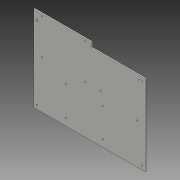
# Autodesk Inventor part: Plate-0
Saved by Autodesk Inventor 2018 (Build 220112000, 112)
## iProperties
Created: 2022-04-19
Part Number: Plate-0
Material: Generic
Document SubType Name: Modeling
Designer: pollak
Density: 1 g/cm^3
Appearance: Default
Author: pollak
Autodesk Inventor part; units mm, degrees
ref_plane "YZ Plane" through (0, 0, 0) normal (1, 0, 0) x (0, 1, 0)
ref_plane "XZ Plane" through (0, 0, 0) normal (0, 1, 0) x (-1, 0, 0)
ref_plane "XY Plane" through (0, 0, 0) normal (0, 0, 1) x (1, 0, 0)
sketch "Sketch1" plane through (0, 0, 0) normal (0, 1, 0) x (-1, 0, 0)
  line L0 (135, 97.5) -> (-135, 97.5)
  line L1 (-135, 97.5) -> (-135, -97.5)
  line L2 (-135, -97.5) -> (135, -97.5)
  line L3 (135, -97.5) -> (135, 97.5)
  line L4 (135, 97.5) -> (-135, -97.5) construction
  line L5 (-135, 97.5) -> (135, -97.5) construction
  line L6 (135, 97.5) -> (-5, 97.5)
  line L7 (-5, 97.5) -> (-5, 109.5)
  line L8 (-5, 109.5) -> (135, 109.5)
  line L9 (135, 109.5) -> (135, 97.5)
  point P0 (0, 0)
  dimension "d0" = 270
  dimension "d1" = 195
  dimension "d2" = 140
  dimension "d3" = 12
  dimension "d4" = 0
  dimension "d5" = 0
  constraints: 20 end point, 4 parallel, 2 horizontal, 2 midpoint, 2 perpendicular
  measures "d0" distance of L2.end L1.end
  measures "d1" distance of L1.end L0.end
  measures "d2" distance of L7.end L8.end
  measures "d3" distance of L6.end L7.end
  measures "d4" distance between parallel lines of L3 L9
  measures "d5" distance between parallel lines of L0 L6
extrude "Extrusion1" add sketch "Sketch1" along normal blind 2.5
sketch "Sketch2" plane through (0, 2.5, 0) normal (0, 1, 0) x (1, 0, 0)
  line L0 (26.75, -17.5) -> (119.25, -17.5) construction
  line L1 (119.25, -17.5) -> (119.25, -87.5) construction
  line L2 (119.25, -87.5) -> (26.75, -87.5) construction
  line L3 (26.75, -87.5) -> (26.75, -17.5) construction
  line L4 (26.75, -17.5) -> (119.25, -87.5) construction
  line L5 (119.25, -17.5) -> (26.75, -87.5) construction
  line L6 (5, -97.5) -> (135, -97.5) construction
  line L7 (135, -97.5) -> (135, 97.5) projected
  point P0 (0, 0)
  point P1 (73, -52.5)
  dimension "d8" = 92.5
  dimension "d9" = 70
  dimension "d10" = 45
  dimension "d11" = 62
  constraints: 12 end point, 2 coincident, 2 midpoint, 2 parallel, 1 horizontal, 1 perpendicular
  measures "d8" distance of L1.end L2.end
  measures "d9" distance of L0.end L1.end
  measures "d10" distance from line of point (73, -52.5) L6
  measures "d11" distance from line of L7 point (73, -52.5)
hole "LRS-35-5" at (26.75, 2.5, 17.5) at (119.25, 2.5, 87.5) direction (0, -1, 0) diameter 2.459 end through all thread size "M3x0.5" class "6H" standard "ISO Metric profile"
sketch "HB12-1.7AG" plane through (0, 2.5, 0) normal (0, 1, 0) x (1, 0, 0)
  line L0 (-115, -103.5) -> (-10.2, -103.5) construction
  line L1 (-10.2, -103.5) -> (-10.2, -17.8) construction
  line L2 (-10.2, -17.8) -> (-115, -17.8) construction
  line L3 (-115, -17.8) -> (-115, -103.5) construction
  line L4 (-115, -103.5) -> (-10.2, -17.8) construction
  line L5 (-10.2, -103.5) -> (-115, -17.8) construction
  line L6 (-135, 97.5) -> (-135, -109.5) construction
  line L7 (-135, -109.5) -> (5, -109.5) construction
  point P0 (0, 0)
  point P1 (-62.6, -60.65)
  dimension "d19" = 104.8
  dimension "d20" = 85.7
  dimension "d23" = 6
  dimension "d24" = 20
  constraints: 12 end point, 4 coincident, 2 midpoint, 2 parallel, 1 horizontal, 1 perpendicular
  measures "d19" distance of L2.end L1.end
  measures "d20" distance of L1.end L0.end
  measures "d23" distance between parallel lines of L0 L7
  measures "d24" distance between parallel lines of L3 L6
hole "BEl PSU" at (-115, 2.5, 17.8) at (-10.2, 2.5, 17.8) at (-10.2, 2.5, 103.5) at (-115, 2.5, 103.5) at (-115, 2.5, 17.8) at (-10.2, 2.5, 17.8) at (-10.2, 2.5, 103.5) at (-115, 2.5, 103.5) direction (0, -1, 0) diameter 2.459 end through all thread size "M3x0.5" class "6H" standard "ISO Metric profile"
sketch "Mounting Holes" plane through (0, 2.5, 0) normal (0, 1, 0) x (1, 0, 0)
  line L0 (-127, -88.9) -> (127, -88.9) construction
  line L1 (127, -88.9) -> (127, 88.9) construction
  line L2 (127, 88.9) -> (-127, 88.9) construction
  line L3 (-127, 88.9) -> (-127, -88.9) construction
  line L4 (-127, -88.9) -> (127, 88.9) construction
  line L5 (127, -88.9) -> (-127, 88.9) construction
  point P0 (0, 0)
  dimension "d32" = 254
  dimension "d33" = 177.8
  constraints: 12 end point, 4 coincident, 2 midpoint, 2 parallel, 1 horizontal, 1 perpendicular
  measures "d32" distance of L2.end L1.end
  measures "d33" distance of L1.end L0.end
hole "Hole3" at (-127, 2.5, -88.9) at (127, 2.5, -88.9) at (127, 2.5, 88.9) at (-127, 2.5, 88.9) direction (0, -1, 0) diameter 4.5 end through all
sketch "WR-LEN" plane through (0, 2.5, 0) normal (0, 1, 0) x (1, 0, 0)
  line L0 (32.5, 80.5) -> (-57.5, 80.5) construction
  line L1 (-57.5, 80.5) -> (-57.5, 10.5) construction
  line L2 (-57.5, 10.5) -> (32.5, 10.5) construction
  line L3 (32.5, 10.5) -> (32.5, 80.5) construction
  line L4 (32.5, 80.5) -> (-57.5, 10.5) construction
  line L5 (-57.5, 80.5) -> (32.5, 10.5) construction
  line L6 (-135, 97.5) -> (-135, -109.5) projected
  line L7 (135, 97.5) -> (-135, 97.5) projected
  point P0 (0, 0)
  point P1 (-12.5, 45.5)
  dimension "d41" = 90
  dimension "d42" = 70
  dimension "d44" = 52
  dimension "d52" = 77.5
  constraints: 12 end point, 4 coincident, 2 midpoint, 2 parallel, 1 horizontal, 1 perpendicular
  measures "d41" distance of L2.end L1.end
  measures "d42" distance of L1.end L0.end
  measures "d44" distance from line of L7 point (-12.5, 45.5)
  measures "d52" distance between parallel lines of L6 L1
hole "WR-LEN-Hole" at (-57.5, 2.5, -80.5) at (32.5, 2.5, -80.5) at (32.5, 2.5, -10.5) at (-57.5, 2.5, -10.5) direction (0, -1, 0) diameter 2.459 end through all thread size "M3x0.5" class "6H" standard "ISO Metric profile"
sketch "GND" plane through (0, 2.5, 0) normal (0, 1, 0) x (1, 0, 0)
  line L0 (135, -97.5) -> (135, 97.5) projected
  line L1 (135, 97.5) -> (-135, 97.5) projected
  point P0 (0, 0)
  point P1 (115, 0)
  dimension "d53" = 20
  dimension "d54" = 97.5
  measures "d53" distance from line of L0 point (115, 0)
  measures "d54" distance from line of L1 point (115, 0)
hole "GND-Hole" at (115, 2.5, 0) direction (0, -1, 0) diameter 3.242 end through all thread size "M4x0.7" class "6H" standard "ISO Metric profile"
body "Solid1"
